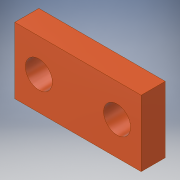
# Autodesk Inventor part: Y-axis Belt clamp
Saved by Autodesk Inventor 2018 (Build 220112000, 112)
## iProperties
Created: 2013-10-27
Part Number: Y-axis Belt clamp
Material: ABS Plastic
Document SubType Name: Modeling
Designer: Gabriel Smolnycki
Mass: 0.844571 g
Surface Area: 7.6748 cm^2
Volume: 0.796765 cm^3
Density: 1.06 g/cm^3
Appearance: Smooth - Light Orange
Author: Gabriel Smolnycki
Sending System: SolidWorks 2017
Last Author: Gabriel Smolnycki
Last Saved: 2017-09-14
Autodesk Inventor part; units mm, degrees
ref_plane "XZ Plane" through (0, 0, 0) normal (0, 1, 0) x (-1, 0, 0)
ref_plane "XY Plane" through (0, 0, 0) normal (0, 0, 1) x (1, 0, 0)
ref_plane "Work Plane1" through (-10.5, 0, 0) normal (1, 0, 0) x (0, 1, 0)
sketch "Sketch1" plane through (-10.5, 0, 0) normal (1, 0, 0) x (0, 1, 0)
  line L0 (5.5, 0) -> (-5.5, 0)
  line L1 (5.5, 4) -> (5.5, 0)
  line L2 (-5.5, 4) -> (-5.5, 0)
  line L3 (5.5, 4) -> (-5.5, 4)
  constraints: 8 end point, 2 horizontal, 2 vertical
extrude "Extrusion1" add sketch "Sketch1" along normal blind 21 draft 0
hole "Hole2" at (6.5, 0, 4) direction (0, 0, -1) diameter 4.5 depth 4 tip angle 118
sketch "Sketch2" plane through (-10.5, -5.5, 4) normal (0, 0, 1) x (1, 0, 0)
  point P0 (17, 5.5)
hole "Hole1" at (-6.5, 0, 4) direction (0, 0, -1) diameter 4.5 depth 4 tip angle 118
sketch "Sketch3" plane through (-10.5, -5.5, 4) normal (0, 0, 1) x (1, 0, 0)
  point P0 (4, 5.5)
body "Solid3"
